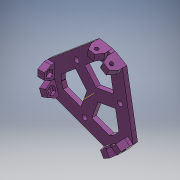
# Autodesk Inventor part: plate_upper
Saved by Autodesk Inventor 2017 (Build 210142000, 142)
## iProperties
Created: 2017-05-06
Part Number: plate_upper
Material: Ogólny
Document SubType Name: Modeling
Designer: Speed King
Density: 1 g/cm^3
Appearance: Gładki - fioletowy
Mass: 14.4594 g
Surface Area: 100.681 cm^2
Volume: 14.4594 cm^3
Author: Speed King
Autodesk Inventor part; units mm, degrees
ref_plane "YZ Plane" through (0, 0, 0) normal (1, 0, 0) x (0, 1, 0)
ref_plane "XZ Plane" through (0, 0, 0) normal (0, 1, 0) x (-1, 0, 0)
sketch "Szkic1" plane through (0, 0, 0) normal (0, 1, 0) x (-1, 0, 0)
  line L0 (70, 0) -> (-70, 0) projected
  line L1 (0, -70) -> (0, 70) projected
  circle A0 centre (0, 0) radius 50
  dimension "d1" = 100
  constraints: 2 midpoint, 1 centre point
  measures "d1" diameter of A0
extrude "Wyciągnięcie proste1" add sketch "Szkic1" along normal blind 4
sketch "Szkic2" plane through (0, 4, 0) normal (0, 1, 0) x (1, 0, 0)
  line L0 (-70, 0) -> (70, 0) projected
  line L1 (-35.15, 6) -> (-41.15, 6)
  line L2 (-41.15, 6) -> (-41.15, -6)
  line L3 (-41.15, -6) -> (-35.15, -6)
  line L4 (-35.15, -6) -> (-35.15, 6)
  line L5 (-35.15, 6) -> (-41.15, -6) construction
  line L6 (-41.15, 6) -> (-35.15, -6) construction
  point P0 (0, 0)
  point P1 (-38.15, 0)
  dimension "d6" = 6
  dimension "d7" = 12
  dimension "d8" = 41.15
  constraints: 12 end point, 2 midpoint, 2 parallel, 1 horizontal, 1 perpendicular, 1 point on line
  measures "d6" distance of L3.end L2.end
  measures "d7" distance of L2.end L1.end
  measures "d8" distance from line of point (0, 0) L2
extrude "Wyciągnięcie proste2" add sketch "Szkic2" against normal blind 13
pattern_circular "Szyk kołowy1" count 2 over 100 about axis through (0, -10, 0) along (0, 1, 0) of "Wyciągnięcie proste2"
pattern_circular "Szyk kołowy2" count 3 over 360 about axis through (0, -10, 0) along (0, 1, 0) of "Wyciągnięcie proste2", "Szyk kołowy1"
sketch "Szkic3" plane through (0, 0, 0) normal (0, -1, 0) x (1, 0, 0)
  line L0 (13.0545, 39.4829) -> (1.2368, 41.5667) projected
  line L1 (25.7712, 32.6369) -> (15.3788, 38.6369) projected
  line L2 (-41.15, 6) -> (-41.15, -6) projected
  line L3 (-40.7205, -8.436) -> (-36.6162, -19.7123) projected
  line L4 (15.3788, -38.6369) -> (25.7712, -32.6369) projected
  line L5 (27.666, -31.047) -> (35.3795, -21.8544) projected
  line L6 (1.2368, 41.5667) -> (13.0545, 39.4829) projected
  line L7 (13.0545, 39.4829) -> (15.3788, 38.6369)
  line L8 (1.2368, 41.5667) -> (-41.15, 6)
  line L9 (-41.15, -6) -> (-40.7205, -8.436)
  line L10 (-36.6162, -19.7123) -> (15.3788, -38.6369)
  line L11 (25.7712, -32.6369) -> (27.666, -31.047)
  line L12 (35.3795, -21.8544) -> (25.7712, 32.6369)
  circle A0 centre (0, 0) radius 50 projected
  constraints: 12 end point, 3 parallel
extrude "Wyciągnięcie proste3" cut sketch "Szkic3" against normal blind 15
sketch "Szkic4" plane through (-41.15, -9, -6) normal (-1, 0, 0) x (0, 0, 1)
  circle A0 centre (6, 4.5) radius 1.7
  line L0 (12, 9) -> (12, 0) projected
  line L1 (0, 9) -> (0, 0) projected
  line L2 (12, 0) -> (0, 0) projected
  line L3 (47.5667, 9) -> (12, 9) projected
  point P0 (6, 9)
  dimension "d19" = 3.4
  dimension "d20" = 12
  dimension "d21" = 9
  dimension "d22" = 4.5
  dimension "d23" = 6
  constraints: 1 centre point
  measures "d19" diameter of A0
  measures "d20" distance between parallel lines of L0 L1
  measures "d21" distance between parallel lines of L2 L3
  measures "d22" distance from line of A0.centre L2
  measures "d23" distance from line of L0 A0.centre
extrude "Wyciągnięcie proste4" cut sketch "Szkic4" against normal blind 15
sketch "Szkic7" plane through (-35.15, -9, 6) normal (1, 0, 0) x (0, 0, -1)
  circle A0 centre (6, 4.5) radius 1.7 projected
  line L0 (4.2102, 7.6) -> (7.7898, 7.6)
  line L1 (7.7898, 7.6) -> (9.5796, 4.5)
  line L2 (9.5796, 4.5) -> (7.7898, 1.4)
  line L3 (7.7898, 1.4) -> (4.2102, 1.4)
  line L4 (4.2102, 1.4) -> (2.4204, 4.5)
  line L5 (2.4204, 4.5) -> (4.2102, 7.6)
  line L6 (27.8544, 9) -> (-26.6369, 9) projected
  point P0 (6, 9)
  dimension "d41" = 6.2
  constraints: 12 end point, 1 coincident, 1 parallel, 13 other
  measures "d41" distance between parallel lines of L3 L0
extrude "Wyciągnięcie proste6" cut sketch "Szkic7" against normal blind 3
sketch "Szkic8" plane through (-41.15, -9, -6) normal (-1, 0, 0) x (0, 0, 1)
  circle A0 centre (6, 4.5) radius 1.7 projected
  line L0 (0, 9) -> (0, 0) projected
  line L1 (12, 0) -> (0, 0) projected
  line L2 (12, 9) -> (12, 0) projected
  line L3 (12, 9) -> (12, 13) projected
  line L4 (0, 13) -> (12, 13) projected
  line L5 (0, 9) -> (0, 13) projected
  line L6 (0, 9) -> (0, 0) projected
  line L7 (0, 6) -> (3, 0)
  line L8 (0, 0) -> (12, 0) projected
  line L9 (6, 13.1218) -> (6, -2.4883) construction
  line L10 (9, 0) -> (12, 6)
  line L11 (12, 9) -> (12, 0) projected
  line L12 (0, 6) -> (0, 0)
  line L13 (0, 0) -> (3, 0)
  line L14 (9, 0) -> (12, 0)
  line L15 (12, 0) -> (12, 6)
  point P0 (6, 9)
  dimension "d44" = 12
  dimension "d45" = 6
  dimension "d46" = 3
  dimension "d47" = 6
  constraints: 14 end point, 4 point on line, 3 collinear, 1 perpendicular, 1 vertical, 1 other
  measures "d44" distance of L4.start L3.end
  measures "d45" distance between parallel lines of L9 L5
  measures "d46" distance of L0.end L7.end
  measures "d47" distance from line of L1 L7.start
extrude "Wyciągnięcie proste7" cut sketch "Szkic8" against normal through all contours L7 L1 L0 | L10 L2 L1
pattern_circular "Szyk kołowy3" count 2 over 100 about axis through (0, -10, 0) along (0, 1, 0) of "Wyciągnięcie proste4", "Wyciągnięcie proste6", "Wyciągnięcie proste7"
pattern_circular "Szyk kołowy4" count 3 over 360 about axis through (0, -10, 0) along (0, 1, 0) of "Wyciągnięcie proste4", "Szyk kołowy3", "Wyciągnięcie proste6", "Wyciągnięcie proste7"
ref_plane "Płaszczyzna konstrukcyjna2" through (0, 0, 0) normal (0.1736, 0, -0.9848) x (0, 1, 0)
ref_plane "Płaszczyzna konstrukcyjna1" through (0, 0, 0) normal (0.9848, 0, 0.1736) x (0, 1, 0)
sketch "Szkic9" plane through (0, 4, 0) normal (0, 1, 0) x (1, 0, 0)
  line L0 (-41.15, -6) -> (1.2368, -41.5667) projected
  line L1 (1.2368, -41.5667) -> (13.0545, -39.4829) projected
  line L2 (13.0545, -39.4829) -> (15.3788, -38.6369) projected
  line L3 (15.3788, -38.6369) -> (25.7712, -32.6369) projected
  line L4 (25.7712, -32.6369) -> (35.3795, 21.8544) projected
  line L5 (35.3795, 21.8544) -> (27.666, 31.047) projected
  line L6 (27.666, 31.047) -> (25.7712, 32.6369) projected
  line L7 (25.7712, 32.6369) -> (15.3788, 38.6369) projected
  line L8 (15.3788, 38.6369) -> (-36.6162, 19.7123) projected
  line L9 (-36.6162, 19.7123) -> (-40.7205, 8.436) projected
  line L10 (-40.7205, 8.436) -> (-41.15, 6) projected
  line L11 (-41.15, 6) -> (-41.15, -6) projected
  line L12 (4.6637, -28.7774) -> (-29.15, -0.4043)
  line L13 (-29.15, -0.4043) -> (-29.15, 4.9501)
  line L14 (-29.15, 4.9501) -> (-29.0851, 5.3183)
  line L15 (-29.0851, 5.3183) -> (-27.2538, 10.3498)
  line L16 (-27.2538, 10.3498) -> (14.2249, 25.4468)
  line L17 (14.2249, 25.4468) -> (18.8619, 22.7696)
  line L18 (18.8619, 22.7696) -> (19.1483, 22.5293)
  line L19 (19.1483, 22.5293) -> (22.5901, 18.4275)
  line L20 (22.5901, 18.4275) -> (14.9251, -25.0425)
  line L21 (14.9251, -25.0425) -> (10.2881, -27.7197)
  line L22 (10.2881, -27.7197) -> (9.9368, -27.8476)
  line L23 (9.9368, -27.8476) -> (4.6637, -28.7774)
  line L24 (-70.5596, 12.4416) -> (63.5408, -11.204) construction
  line L25 (0, 0) -> (-18.2691, 50.194) construction
  line L26 (0, 0) -> (-31.1455, -37.1177) construction
  line L27 (17.8412, -8.5048) -> (2.0843, -5.7264)
  line L28 (2.0843, -5.7264) -> (-8.2003, -17.9832)
  line L29 (-16.286, -11.1985) -> (-6.0014, 1.0582)
  line L30 (19.674, 1.8899) -> (3.9171, 4.6682)
  line L31 (3.9171, 4.6682) -> (-1.5552, 19.7033)
  line L32 (-6.0014, 1.0582) -> (-11.4737, 16.0933)
  line L33 (0, 0) -> (30.8041, 36.7109) construction
  line L34 (0, 0) -> (16.6908, -45.8576) construction
  dimension "d50" = 12
  dimension "d51" = 120
  dimension "d52" = 120
  dimension "d54" = 16
  dimension "d55" = 16
  constraints: 44 end point, 9 point on line, 6 perpendicular, 2 collinear, 12 other
  measures "d50" distance between parallel lines of L0 L12
  measures "d51" angle of L25 L24
  measures "d52" angle of L26 L25
  measures "d54" distance of L30.start L30.end
  measures "d55" distance of L29.end L32.end
extrude "Wyciągnięcie proste8" cut sketch "Szkic9" against normal blind 10 contours L12 L28 L27 L20 L21 L22 L23 | L12 L13 L14 L15 L16 L32 L29 | L30 L31 L16 L17 L18 L19 L20
sketch "Szkic10" plane through (0, 4, 0) normal (0, 1, 0) x (1, 0, 0)
  line L0 (0, 0) -> (32.0857, 38.2383) construction
  line L1 (0, 0) -> (16.7031, -45.8915) construction
  line L2 (-64.2519, 11.3293) -> (59.8959, -10.5613) construction
  circle A0 centre (-8.2085, 22.5526) radius 2.25
  circle A1 centre (23.6354, -4.1676) radius 2.25
  circle A2 centre (-15.4269, -18.3851) radius 2.25
  dimension "d58" = 120
  dimension "d59" = 120
  dimension "d68" = 4.5
  dimension "d69" = 4.5
  dimension "d70" = 4.5
  dimension "d71" = 24
  dimension "d72" = 24
  dimension "d73" = 24
  constraints: 4 end point, 3 centre point, 3 point on line
  measures "d58" angle of L0 L2
  measures "d59" angle of L1 L0
  measures "d68" diameter of A0
  measures "d69" diameter of A2
  measures "d70" diameter of A1
  measures "d71" distance of A0.centre L0.start
  measures "d72" distance of L0.start A2.centre
  measures "d73" distance of A1.centre L0.start
extrude "Wyciągnięcie proste9" cut sketch "Szkic10" against normal blind 10
equation "\"d8\" = radiusPlatform - ballOffset"
equation "\"d12\" = alphaPlatform"
equation "\"d22\" = 0.5 * d21"
equation "\"d23\" = 0.5 * d20"
equation "\"d45\" = 0.5 * d44"
equation "\"d27\" = alphaPlatform"
equation "\"d55\" = d54"
equation "\"d69\" = d68"
equation "\"d70\" = d68"
equation "\"d72\" = d71"
equation "\"d73\" = d71"
equation "\"alphaPlatform\" = 100deg"
equation "\"radiusPlatform\" = 50"
equation "\"ballOffset\" = 8.85"
